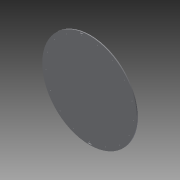
# Autodesk Inventor part: laser circle3d back
Saved by Autodesk Inventor 2013 (Build 170138000, 138)
## iProperties
Created: 2013-07-18
Part Number: laser circle3d back
Material: Generic
Document SubType Name: Modeling
Designer: owner
Density: 1 g/cm^3
Author: owner
Autodesk Inventor part; units mm, degrees
ref_plane "YZ Plane" through (0, 0, 0) normal (1, 0, 0) x (0, 1, 0)
ref_plane "XZ Plane" through (0, 0, 0) normal (0, 1, 0) x (-1, 0, 0)
ref_plane "XY Plane" through (0, 0, 0) normal (0, 0, 1) x (1, 0, 0)
sketch "Sketch1" plane through (0, 0, 0) normal (0, 0, 1) x (1, 0, 0)
  circle A0 centre (0, 0) radius 355.6
  circle A1 centre (0, -330.2) radius 3.175
  circle A2 centre (119.282, -307.9023) radius 3.175
  circle A3 centre (222.4543, -244.0207) radius 3.175
  circle A4 centre (295.5829, -147.1828) radius 3.175
  circle A5 centre (328.7914, -30.467) radius 3.175
  circle A6 centre (317.5948, 90.3635) radius 3.175
  circle A7 centre (263.5053, 198.99) radius 3.175
  circle A8 centre (173.8279, 280.7417) radius 3.175
  circle A9 centre (60.6741, 324.5777) radius 3.175
  circle A10 centre (-60.6741, 324.5777) radius 3.175
  circle A11 centre (-173.8279, 280.7417) radius 3.175
  circle A12 centre (-263.5053, 198.99) radius 3.175
  circle A13 centre (-317.5948, 90.3635) radius 3.175
  circle A14 centre (-328.7914, -30.467) radius 3.175
  circle A15 centre (-295.5829, -147.1828) radius 3.175
  circle A16 centre (-222.4543, -244.0207) radius 3.175
  circle A17 centre (-119.282, -307.9023) radius 3.175
  line L0 (0, -342.9) -> (12.7, -342.9)
  line L1 (12.7, -342.9) -> (12.7, -349.25)
  line L2 (12.7, -349.25) -> (-12.7, -349.25)
  line L3 (-12.7, -349.25) -> (-12.7, -342.9)
  line L4 (-12.7, -342.9) -> (0, -342.9)
  line L5 (-75.5018, 334.7255) -> (-76.6688, 340.9674)
  line L6 (-63.0181, 337.0595) -> (-75.5018, 334.7255)
  line L7 (-50.5344, 339.3935) -> (-63.0181, 337.0595)
  line L8 (-76.6688, 340.9674) -> (-51.7014, 345.6354)
  line L9 (-51.7014, 345.6354) -> (-50.5344, 339.3935)
  dimension "d0" = 711.2
  dimension "d2" = 6.35
  dimension "d5" = 360
  dimension "d7" = 12.7
  dimension "d8" = 6.35
  dimension "d9" = 25.4
  constraints: 20 end point, 18 centre point, 1 coincident, 1 collinear, 1 parallel, 35 other
  measures "d0" diameter of A0
  measures "d2" diameter of A1
  measures "d7" distance of L0.start L0.end
  measures "d8" distance of L0.end L1.end
  measures "d9" distance of L1.end L3.start
extrude "Extrusion1" add sketch "Sketch1" along normal blind 6.35
body "Solid1"
